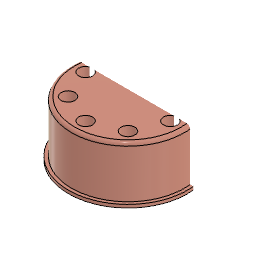
CarrierOutput (Autodesk Fusion 360 design; units mm, degrees)
Autodesk Fusion 360 part; units mm, degrees
sketch "Carrier" plane through (0, 0, 0) normal (0, 0, 1) x (1, 0, 0)
  circle A0 centre (0, 0) radius 17.55
  circle A1 centre (0, 0) radius 18.55
  dimension "d256" = 35.1
  dimension "d259" = 1
  constraint coincident A0.centre A1.centre
  measures "d256" diameter of A0
extrude "Extrude31" add sketch "Carrier" along normal blind 17 contours A0
extrude "Extrude32" add sketch "Carrier" along normal blind 1
fillet "Fillet12" radius 1 1 edges at (-16.3623, -6.3464, 17)
sketch "heat inserts" plane through (0, 0, 17) normal (0, 0, 1) x (-1, 0, 0)
  circle A0 centre (0, 0) radius 16.55
  line L0 (0, 0) -> (0, -13.2) construction
  circle A1 centre (0, -13.2) radius 2.15
  dimension "d264" = 13.2
  dimension "d265" = 4.3
  constraint vertical L0
  constraint coincident A0.centre L0.start
  constraint coincident L0.end A1.centre
  measures "d264" distance of A0.centre L0.end
  measures "d265" diameter of A1
extrude "Extrude33" cut sketch "heat inserts" against normal blind 12 contours A1
pattern_circular "C-Pattern7" count 8 over 360 about axis through (0, 0, 17) along (0, 0, -1) of "Extrude33"
equation "bearing_mount_lip = 1 mm"
equation "m3 = 3.05 mm"
equation "heat_insert_diameter = 4.3 mm"
equation "output_bearing_id = 35 mm"
equation "heat_insert_distance = ( output_bearing_id / 2 ) - heat_insert_diameter"
equation "n_heat_insert = 8"
equation "height = 17 mm"
equation "heat_insert_depth = 12 mm"
equation "d256 = output_bearing_id + bearing_id_fit"
equation "d257 = height"
equation "d260 = bearing_mount_lip"
equation "d264 = heat_insert_distance"
equation "d265 = heat_insert_diameter"
equation "d266 = -heat_insert_depth"
equation "d268 = n_heat_insert"
equation "bearing_id_fit = 0.1 mm"
